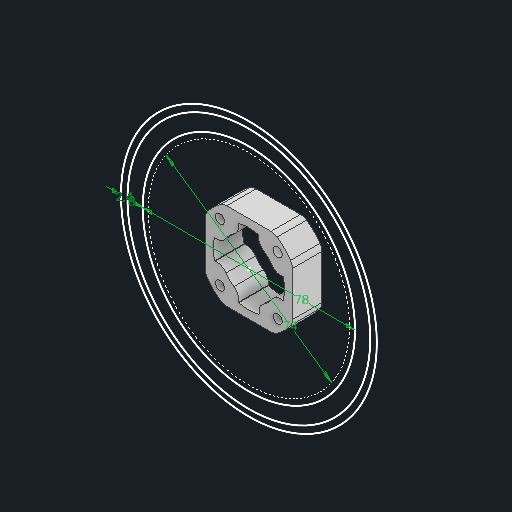
# Autodesk Inventor part: Test_block
Saved by Autodesk Inventor 2025.1 (Build 291241020, 241B)
## iProperties
Created: 2025-07-24
Part Number: Test_block
Material: 일반
Document SubType Name: Modeling
Designer: acalo
Density: 1 g/cm^3
Appearance: 기본값
Author: acalo
Autodesk Inventor part; units mm, degrees
ref_plane "YZ Plane" through (0, 0, 0) normal (1, 0, 0) x (0, 1, 0)
ref_plane "XZ Plane" through (0, 0, 0) normal (0, 1, 0) x (-1, 0, 0)
ref_plane "XY Plane" through (0, 0, 0) normal (0, 0, 1) x (1, 0, 0)
sketch "스케치1" plane through (0, 0, 0) normal (0, 0, 1) x (1, 0, 0)
  arc A0 (-1.5318, 18.4365) -> (1.5318, 18.4365) centre (0, 0) ccw
  circle A1 centre (10.6066, -10.6066) radius 1.65
  circle A2 centre (-10.6066, 10.6066) radius 1.65
  arc A3 (-12.137, 5.5852) -> (-14.408, 4.1723) centre (-12.487, 3.616) ccw
  arc A4 (-12.137, 5.5852) -> (-10.1031, 6.4751) centre (-11.787, 7.5543) ccw
  arc A5 (-6.5731, 10.0397) -> (-10.1031, 6.4751) centre (0, 0) ccw
  arc A6 (-6.5731, 10.0397) -> (-5.7029, 12.0821) centre (-7.6686, 11.7129) ccw
  arc A7 (-4.3123, 14.3668) -> (-5.7029, 12.0821) centre (-3.7373, 12.4512) ccw
  arc A8 (4.1723, 14.408) -> (-4.3123, 14.3668) centre (0, 0) ccw
  arc A9 (5.5852, 12.137) -> (4.1723, 14.408) centre (3.616, 12.487) ccw
  arc A10 (5.5852, 12.137) -> (6.4751, 10.1031) centre (7.5543, 11.787) ccw
  arc A11 (10.0397, 6.5731) -> (6.4751, 10.1031) centre (0, 0) ccw
  arc A12 (10.0397, 6.5731) -> (12.0821, 5.7029) centre (11.7129, 7.6686) ccw
  arc A13 (14.3668, 4.3123) -> (12.0821, 5.7029) centre (12.4512, 3.7373) ccw
  arc A14 (14.408, -4.1723) -> (14.3668, 4.3123) centre (0, 0) ccw
  arc A15 (12.137, -5.5852) -> (14.408, -4.1723) centre (12.487, -3.616) ccw
  arc A16 (12.137, -5.5852) -> (10.1031, -6.4751) centre (11.787, -7.5543) ccw
  arc A17 (6.5731, -10.0397) -> (10.1031, -6.4751) centre (0, 0) ccw
  arc A18 (6.5731, -10.0397) -> (5.7029, -12.0821) centre (7.6686, -11.7129) ccw
  arc A19 (4.3123, -14.3668) -> (5.7029, -12.0821) centre (3.7373, -12.4512) ccw
  arc A20 (-4.1723, -14.408) -> (4.3123, -14.3668) centre (0, 0) ccw
  arc A21 (-5.5852, -12.137) -> (-4.1723, -14.408) centre (-3.616, -12.487) ccw
  arc A22 (-5.5852, -12.137) -> (-6.4751, -10.1031) centre (-7.5543, -11.787) ccw
  arc A23 (-10.0397, -6.5731) -> (-6.4751, -10.1031) centre (0, 0) ccw
  arc A24 (-10.0397, -6.5731) -> (-12.0821, -5.7029) centre (-11.7129, -7.6686) ccw
  arc A25 (-14.3668, -4.3123) -> (-12.0821, -5.7029) centre (-12.4512, -3.7373) ccw
  arc A26 (-14.408, 4.1723) -> (-14.3668, -4.3123) centre (0, 0) ccw
  circle A27 centre (-10.6066, -10.6066) radius 1.65
  circle A28 centre (10.6066, 10.6066) radius 1.65
  circle A29 centre (0, 0) radius 18.5
  point P0 (0, 0)
  point P1 (0, 0)
  point P2 (1.5318, 18.4365)
  point P3 (-1.5318, 18.4365)
  constraints: 50 point on circle, 30 centre point, 1 coincident
extrude "돌출1" add sketch "스케치1" along normal blind 10.8
sketch "스케치2" plane through (0, 0, 0) normal (0, 0, -1) x (-1, 0, 0)
  circle A0 centre (0, 0) radius 10
  circle A1 centre (0, 0) radius 18.5
  circle A2 centre (-10.6066, 10.6066) radius 1.65
  circle A3 centre (10.6066, -10.6066) radius 1.65
  arc A4 (5.8013, 12.0816) -> (6.5731, 10.0397) centre (7.7549, 11.6531) ccw
  arc A5 (10.1031, 6.4751) -> (6.5731, 10.0397) centre (0, 0) ccw
  arc A6 (10.1031, 6.4751) -> (12.137, 5.5852) centre (11.787, 7.5543) ccw
  arc A7 (14.5614, 3.9084) -> (12.137, 5.5852) centre (12.558, 3.6028) ccw
  arc A8 (14.428, -4.275) -> (14.5614, 3.9084) centre (0.0099, 0.0527) ccw
  arc A9 (12.0821, -5.7029) -> (14.428, -4.275) centre (12.4611, -3.6846) ccw
  arc A10 (12.0821, -5.7029) -> (10.0397, -6.5731) centre (11.7129, -7.6686) ccw
  arc A11 (6.4751, -10.1031) -> (10.0397, -6.5731) centre (0, 0) ccw
  arc A12 (6.4751, -10.1031) -> (5.687, -12.1375) centre (7.6442, -11.7259) ccw
  arc A13 (4.2376, -14.4673) -> (5.687, -12.1375) centre (3.6669, -12.4965) ccw
  arc A14 (-4.2763, -14.4259) -> (4.2376, -14.4673) centre (0.0509, -0.0096) ccw
  arc A15 (-5.7029, -12.0821) -> (-4.2763, -14.4259) centre (-3.6864, -12.4608) ccw
  arc A16 (-5.7029, -12.0821) -> (-6.5731, -10.0397) centre (-7.6686, -11.7129) ccw
  arc A17 (-10.1031, -6.4751) -> (-6.5731, -10.0397) centre (0, 0) ccw
  arc A18 (-10.1031, -6.4751) -> (-12.1375, -5.6835) centre (-11.728, -7.6412) ccw
  arc A19 (-14.4653, -4.2354) -> (-12.1375, -5.6835) centre (-12.4962, -3.6652) ccw
  arc A20 (-14.4239, 4.2775) -> (-14.4653, -4.2354) centre (-0.0092, -0.0491) ccw
  arc A21 (-12.0821, 5.7029) -> (-14.4239, 4.2775) centre (-12.4604, 3.6882) ccw
  arc A22 (-12.0821, 5.7029) -> (-10.0397, 6.5731) centre (-11.7129, 7.6686) ccw
  arc A23 (-6.4751, 10.1031) -> (-10.0397, 6.5731) centre (0, 0) ccw
  arc A24 (-6.4751, 10.1031) -> (-5.5852, 12.137) centre (-7.5543, 11.787) ccw
  arc A25 (-4.137, 14.4648) -> (-5.5852, 12.137) centre (-3.5668, 12.4957) ccw
  arc A26 (4.3759, 14.4234) -> (-4.137, 14.4648) centre (0.0492, 0.0087) ccw
  arc A27 (5.8013, 12.0816) -> (4.3759, 14.4234) centre (3.7865, 12.46) ccw
  circle A28 centre (10.6066, 10.6066) radius 1.65
  circle A29 centre (-10.6066, -10.6066) radius 1.65
  arc A30 (-12.442, 3.7864) -> (-8.4082, 5.5049) centre (-11.7129, 7.6686) ccw
  arc A31 (-12.442, 3.7864) -> (-12.5562, 3.7169) centre (-12.4604, 3.6882) ccw
  arc A32 (-12.5562, 3.7169) -> (-12.5923, -3.693) centre (-0.0092, -0.0491) ccw
  arc A33 (-12.5923, -3.693) -> (-12.4787, -3.7636) centre (-12.4962, -3.6652) ccw
  arc A34 (-8.4028, -5.51) -> (-12.4787, -3.7636) centre (-11.728, -7.6412) ccw
  arc A35 (-8.4028, -5.51) -> (-5.504, -8.4067) centre (0, 0) ccw
  arc A36 (-3.7847, -12.4423) -> (-5.504, -8.4067) centre (-7.6686, -11.7129) ccw
  arc A37 (-3.7847, -12.4423) -> (-3.7152, -12.5565) centre (-3.6864, -12.4608) ccw
  arc A38 (-3.7152, -12.5565) -> (3.6947, -12.5926) centre (0.0509, -0.0096) ccw
  arc A39 (3.6947, -12.5926) -> (3.7653, -12.479) centre (3.6669, -12.4965) ccw
  arc A40 (5.5121, -8.3992) -> (3.7653, -12.479) centre (7.6442, -11.7259) ccw
  arc A41 (5.5121, -8.3992) -> (8.4052, -5.503) centre (0, 0) ccw
  arc A42 (12.4426, -3.7829) -> (8.4052, -5.503) centre (11.7129, -7.6686) ccw
  arc A43 (12.4426, -3.7829) -> (12.5569, -3.7133) centre (12.4611, -3.6846) ccw
  arc A44 (12.5569, -3.7133) -> (12.5929, 3.6965) centre (0.0099, 0.0527) ccw
  arc A45 (12.5929, 3.6965) -> (12.4785, 3.6635) centre (12.558, 3.6028) ccw
  arc A46 (8.4599, 5.422) -> (12.4785, 3.6635) centre (11.787, 7.5543) ccw
  arc A47 (8.4599, 5.422) -> (5.5915, 8.3488) centre (0, 0) ccw
  arc A48 (3.8848, 12.4415) -> (5.5915, 8.3488) centre (7.7549, 11.6531) ccw
  arc A49 (3.8848, 12.4415) -> (3.8153, 12.5557) centre (3.7865, 12.46) ccw
  arc A50 (3.8153, 12.5557) -> (-3.5946, 12.5918) centre (0.0492, 0.0087) ccw
  arc A51 (-3.5946, 12.5918) -> (-3.6652, 12.4782) centre (-3.5668, 12.4957) ccw
  arc A52 (-5.4229, 8.4614) -> (-3.6652, 12.4782) centre (-7.5543, 11.787) ccw
  arc A53 (-5.4229, 8.4614) -> (-8.4082, 5.5049) centre (0, 0) ccw
  point P0 (-8.45, 5.5323)
  point P1 (-5.4499, 8.5035)
  point P2 (5.5323, 8.45)
  point P3 (8.5035, 5.4499)
  point P4 (8.45, -5.5323)
  point P5 (5.4499, -8.5035)
  point P6 (-5.5323, -8.45)
  point P7 (-8.5035, -5.4499)
  dimension "d2" = 20
  dimension "d3" = 1.95
  constraints: 96 point on circle, 82 centre point, 1 coincident, 4 other
  measures "d2" diameter of A0
  measures "d3" radial gap between concentric circles of A23 A53
extrude "돌출2" add sketch "스케치2" against normal up to surface (10.8 mm away) contours A4 A5 A6 A7 A8 A9 A10 A11 A12 A13 A14 A15 A16 A17 A18 A19 A20 A21 A22 A23 A24 A25 A26 A27
sketch "스케치3" plane through (0, 0, 0) normal (0, 0, -1) x (-1, 0, 0)
  line L0 (-16, 16) -> (16, 16)
  line L1 (16, 16) -> (16, -16)
  line L2 (16, -16) -> (-16, -16)
  line L3 (-16, -16) -> (-16, 16)
  line L4 (-16, 16) -> (16, -16) construction
  line L5 (16, 16) -> (-16, -16) construction
  circle A0 centre (0, 0) radius 18.5 projected
  circle A1 centre (-10.6066, 10.6066) radius 1.65 projected
  circle A2 centre (10.6066, -10.6066) radius 1.65 projected
  circle A3 centre (10.6066, 10.6066) radius 1.65 projected
  circle A4 centre (-10.6066, -10.6066) radius 1.65 projected
  point P0 (0, 0)
  point P1 (-9.2871, -16)
  point P2 (9.2871, -16)
  point P3 (16, 9.2871)
  point P4 (16, -9.2871)
  point P5 (9.2871, 16)
  point P6 (-9.2871, 16)
  point P7 (-16, 9.2871)
  point P8 (-16, -9.2871)
  dimension "d6" = 32
  dimension "d7" = 32
  constraints: 12 end point, 2 midpoint, 2 parallel, 1 horizontal, 1 perpendicular
  measures "d6" distance of L1.end L2.end
  measures "d7" distance of L0.end L1.end
extrude "돌출3" cut sketch "스케치3" against normal through all contours A0 L0 | L3 A0 | A0 L1 | L2 A0
fillet "모깎기1" radius 4 8 edges at (16, 9.2871, 5.4) (16, -9.2871, 5.4) (9.2871, 16, 5.4) (-9.2871, 16, 5.4) (9.2871, -16, 5.4) (-9.2871, -16, 5.4) (-16, 9.2871, 5.4) (-16, -9.2871, 5.4)
sketch "스케치4" plane through (0, 0, 10.8) normal (0, 0, 1) x (1, 0, 0)
  circle A0 centre (0, 0) radius 39
  circle A1 centre (0, 0) radius 37 construction
  circle A2 centre (0, 0) radius 47
  circle A3 centre (0, 0) radius 44.6
  dimension "d11" = 78
  dimension "d12" = 74
  dimension "d13" = 8
  dimension "d14" = 2.4
  constraints: 4 centre point, 2 coincident
  measures "d11" diameter of A0
  measures "d12" diameter of A1
  measures "d13" radial gap between concentric circles of A0 A2
  measures "d14" radial gap between concentric circles of A2 A3
